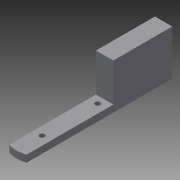
# Autodesk Inventor part: Valve
Saved by Autodesk Inventor 2015 (Build 190159000, 159)
## iProperties
Created: 2016-01-09
Part Number: Valve
Material: Generic
Document SubType Name: Modeling
Designer: HP USER
Density: 1 g/cm^3
Appearance: Default
Author: HP USER
Autodesk Inventor part; units mm, degrees
ref_plane "YZ Plane" through (0, 0, 0) normal (1, 0, 0) x (0, 1, 0)
ref_plane "XZ Plane" through (0, 0, 0) normal (0, 1, 0) x (-1, 0, 0)
ref_plane "XY Plane" through (0, 0, 0) normal (0, 0, 1) x (1, 0, 0)
sketch "Sketch1" plane through (0, 0, 0) normal (0, 0, 1) x (1, 0, 0)
  line L0 (-2.5, -35.0001) -> (2.5, -35.0001)
  line L1 (2.8921, 7.4595) -> (4.1309, 9.1069)
  line L2 (-2.8882, 7.4611) -> (-3.0825, 9.5131)
  line L3 (-3.0825, 9.5131) -> (-5.3884, 5.9139)
  line L4 (-5.3884, 5.9139) -> (-6.3108, 7.7572)
  line L5 (-6.3108, 7.7572) -> (-7.1609, 3.5681)
  line L6 (-7.1609, 3.5681) -> (-8.6869, 4.9536)
  line L7 (-8.6869, 4.9536) -> (-7.9662, 0.7403)
  line L8 (-7.9662, 0.7403) -> (-9.8897, 1.481)
  line L9 (-9.8897, 1.481) -> (-7.6957, -2.1874)
  line L10 (-7.6957, -2.1874) -> (-9.7569, -2.1916)
  line L11 (-9.7569, -2.1916) -> (-6.3859, -4.8197)
  line L12 (-6.3859, -4.8197) -> (-8.3064, -5.5682)
  line L13 (-8.3064, -5.5682) -> (-4.2136, -6.8011)
  line L14 (-4.2136, -6.8011) -> (-5.734, -8.1928)
  line L15 (-5.734, -8.1928) -> (-1.4722, -7.864)
  line L16 (-1.4722, -7.864) -> (-2.3872, -9.7109)
  line L17 (-2.3872, -9.7109) -> (1.468, -7.8647)
  line L18 (1.468, -7.8647) -> (1.282, -9.9175)
  line L19 (1.282, -9.9175) -> (4.21, -6.8033)
  line L20 (4.21, -6.8033) -> (4.778, -8.7847)
  line L21 (4.778, -8.7847) -> (6.3833, -4.8231)
  line L22 (6.3833, -4.8231) -> (7.6287, -6.4655)
  line L23 (7.6287, -6.4655) -> (7.6946, -2.1915)
  line L24 (7.6946, -2.1915) -> (9.4492, -3.273)
  line L25 (9.4492, -3.273) -> (7.9666, 0.7361)
  line L26 (7.9666, 0.7361) -> (9.9935, 0.3614)
  line L27 (9.9935, 0.3614) -> (7.1628, 3.5643)
  line L28 (7.1628, 3.5643) -> (9.1881, 3.9471)
  line L29 (9.1881, 3.9471) -> (5.3915, 5.9111)
  line L30 (5.3915, 5.9111) -> (7.1418, 6.9996)
  line L31 (7.1418, 6.9996) -> (2.8921, 7.4595)
  line L32 (-2.5, -35) -> (2.5, -35)
  line L33 (2.5, 35) -> (-2.5, 35)
  arc A0 (-2.5, -7.011) -> (2.5, -7.011) centre (0, 0) ccw
  line L34 (2.5, -7.011) -> (2.5, 35)
  line L35 (-2.5, 35) -> (-2.5, -7.011)
  circle A1 centre (0, 16) radius 0.75
  circle A2 centre (0, 0) radius 0.75
  dimension "d3" = 5
  dimension "d5" = 1.5
  dimension "d6" = 1.5
  constraints: 72 end point, 3 centre point, 2 horizontal, 2 parallel, 2 point on circle, 1 coincident, 1 perpendicular
  measures "d3" distance of L33.end L33.start
  measures "d5" diameter of A1
  measures "d6" diameter of A2
extrude "Extrusion1" add sketch "Sketch1" along normal blind 2
sketch "Sketch2" plane through (0, 0, 2) normal (0, 0, 1) x (1, 0, 0)
  circle A0 centre (0, 0) radius 0.75 projected
  line L0 (2.5, 18) -> (2.5, 35)
  line L1 (2.5, 35) -> (-2.5, 35)
  line L2 (-2.5, 35) -> (-2.5, 18)
  line L3 (2.5, 18) -> (-2.5, 18)
  line L4 (-2.5, 35) -> (-2.5, -7.011) projected
  constraints: 8 end point, 1 parallel, 1 perpendicular, 1 point on line
extrude "Extrusion2" add sketch "Sketch2" along normal blind 11 contours L3 L2 L1 L0
body "Solid1"
